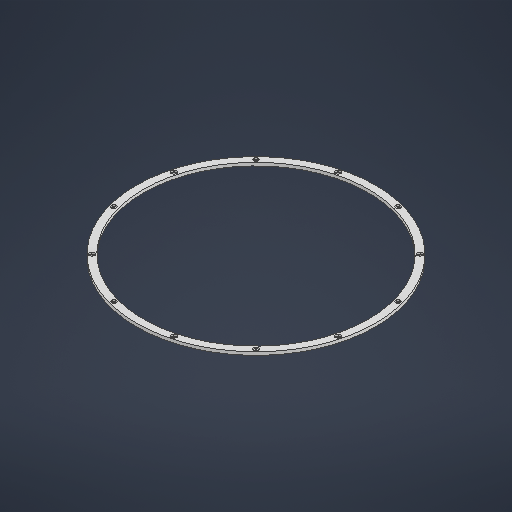
# Autodesk Inventor part: ArmLoopOuterRing
Saved by Autodesk Inventor 2026.1 (Build 301233020, 233B)
## iProperties
Created: 2025-10-19
Part Number: ArmLoopOuterRing
Material: Generic
Document SubType Name: Modeling
Designer: skybound
Density: 1 g/cm^3
Appearance: Default
Author: skybound
Autodesk Inventor part; units mm, degrees
ref_plane "YZ Plane" through (0, 0, 0) normal (1, 0, 0) x (0, 1, 0)
ref_plane "XZ Plane" through (0, 0, 0) normal (0, 1, 0) x (-1, 0, 0)
ref_plane "XY Plane" through (0, 0, 0) normal (0, 0, 1) x (1, 0, 0)
sketch "Sketch1" plane through (0, 0, 0) normal (0, 1, 0) x (-1, 0, 0)
  circle A0 centre (0, 0) radius 144.3
  circle A1 centre (0, 0) radius 153.3
  dimension "d1" = 9
  dimension "d5" = 306.6
  constraints: 2 centre point, 1 coincident
  measures "d1" radial gap between concentric circles of A0 A1
  measures "d5" diameter of A1
extrude "Extrusion1" add sketch "Sketch1" along normal blind 4
sketch "Sketch2" plane through (0, 4, 0) normal (0, 1, 0) x (1, 0, 0)
  line L0 (0, 0) -> (143.7298, 38.5123) construction
  line L1 (146.1384, 40.9209) -> (147.0201, 37.6306)
  line L2 (147.0201, 37.6306) -> (144.6114, 35.222)
  line L3 (144.6114, 35.222) -> (141.3211, 36.1036)
  line L4 (141.3211, 36.1036) -> (140.4395, 39.3939)
  line L5 (140.4395, 39.3939) -> (142.8481, 41.8026)
  line L6 (142.8481, 41.8026) -> (146.1384, 40.9209)
  line L7 (0, 0) -> (153.3, 0) construction
  circle A0 centre (0, 0) radius 153.3 projected
  line L8 (102.8088, 107.6262) -> (106.0991, 108.5078)
  line L9 (101.9272, 104.3359) -> (102.8088, 107.6262)
  line L10 (104.3359, 101.9272) -> (101.9272, 104.3359)
  line L11 (107.6262, 102.8088) -> (104.3359, 101.9272)
  line L12 (108.5078, 106.0991) -> (107.6262, 102.8088)
  line L13 (106.0991, 108.5078) -> (108.5078, 106.0991)
  line L14 (35.222, 144.6114) -> (37.6306, 147.0201)
  line L15 (36.1036, 141.3211) -> (35.222, 144.6114)
  line L16 (39.3939, 140.4395) -> (36.1036, 141.3211)
  line L17 (41.8026, 142.8481) -> (39.3939, 140.4395)
  line L18 (40.9209, 146.1384) -> (41.8026, 142.8481)
  line L19 (37.6306, 147.0201) -> (40.9209, 146.1384)
  line L20 (-41.8026, 142.8481) -> (-40.9209, 146.1384)
  line L21 (-39.3939, 140.4395) -> (-41.8026, 142.8481)
  line L22 (-36.1036, 141.3211) -> (-39.3939, 140.4395)
  line L23 (-35.222, 144.6114) -> (-36.1036, 141.3211)
  line L24 (-37.6306, 147.0201) -> (-35.222, 144.6114)
  line L25 (-40.9209, 146.1384) -> (-37.6306, 147.0201)
  line L26 (-107.6262, 102.8088) -> (-108.5078, 106.0991)
  line L27 (-104.3359, 101.9272) -> (-107.6262, 102.8088)
  line L28 (-101.9272, 104.3359) -> (-104.3359, 101.9272)
  line L29 (-102.8088, 107.6262) -> (-101.9272, 104.3359)
  line L30 (-106.0991, 108.5078) -> (-102.8088, 107.6262)
  line L31 (-108.5078, 106.0991) -> (-106.0991, 108.5078)
  line L32 (-144.6114, 35.222) -> (-147.0201, 37.6306)
  line L33 (-141.3211, 36.1036) -> (-144.6114, 35.222)
  line L34 (-140.4395, 39.3939) -> (-141.3211, 36.1036)
  line L35 (-142.8481, 41.8026) -> (-140.4395, 39.3939)
  line L36 (-146.1384, 40.9209) -> (-142.8481, 41.8026)
  line L37 (-147.0201, 37.6306) -> (-146.1384, 40.9209)
  line L38 (-142.8481, -41.8026) -> (-146.1384, -40.9209)
  line L39 (-140.4395, -39.3939) -> (-142.8481, -41.8026)
  line L40 (-141.3211, -36.1036) -> (-140.4395, -39.3939)
  line L41 (-144.6114, -35.222) -> (-141.3211, -36.1036)
  line L42 (-147.0201, -37.6306) -> (-144.6114, -35.222)
  line L43 (-146.1384, -40.9209) -> (-147.0201, -37.6306)
  line L44 (-102.8088, -107.6262) -> (-106.0991, -108.5078)
  line L45 (-101.9272, -104.3359) -> (-102.8088, -107.6262)
  line L46 (-104.3359, -101.9272) -> (-101.9272, -104.3359)
  line L47 (-107.6262, -102.8088) -> (-104.3359, -101.9272)
  line L48 (-108.5078, -106.0991) -> (-107.6262, -102.8088)
  line L49 (-106.0991, -108.5078) -> (-108.5078, -106.0991)
  line L50 (-35.222, -144.6114) -> (-37.6306, -147.0201)
  line L51 (-36.1036, -141.3211) -> (-35.222, -144.6114)
  line L52 (-39.3939, -140.4395) -> (-36.1036, -141.3211)
  line L53 (-41.8026, -142.8481) -> (-39.3939, -140.4395)
  line L54 (-40.9209, -146.1384) -> (-41.8026, -142.8481)
  line L55 (-37.6306, -147.0201) -> (-40.9209, -146.1384)
  line L56 (41.8026, -142.8481) -> (40.9209, -146.1384)
  line L57 (39.3939, -140.4395) -> (41.8026, -142.8481)
  line L58 (36.1036, -141.3211) -> (39.3939, -140.4395)
  line L59 (35.222, -144.6114) -> (36.1036, -141.3211)
  line L60 (37.6306, -147.0201) -> (35.222, -144.6114)
  line L61 (40.9209, -146.1384) -> (37.6306, -147.0201)
  line L62 (107.6262, -102.8088) -> (108.5078, -106.0991)
  line L63 (104.3359, -101.9272) -> (107.6262, -102.8088)
  line L64 (101.9272, -104.3359) -> (104.3359, -101.9272)
  line L65 (102.8088, -107.6262) -> (101.9272, -104.3359)
  line L66 (106.0991, -108.5078) -> (102.8088, -107.6262)
  line L67 (108.5078, -106.0991) -> (106.0991, -108.5078)
  line L68 (144.6114, -35.222) -> (147.0201, -37.6306)
  line L69 (141.3211, -36.1036) -> (144.6114, -35.222)
  line L70 (140.4395, -39.3939) -> (141.3211, -36.1036)
  line L71 (142.8481, -41.8026) -> (140.4395, -39.3939)
  line L72 (146.1384, -40.9209) -> (142.8481, -41.8026)
  line L73 (147.0201, -37.6306) -> (146.1384, -40.9209)
  dimension "d6" = 148.8
  dimension "d7" = 5.9
  dimension "d8" = 15
  dimension "d11" = 360
  constraints: 148 end point, 1 coincident, 1 horizontal, 1 horizontal alignment, 1 perpendicular, 159 other
  measures "d6" distance of L0.start L0.end
  measures "d7" distance between parallel lines of L1 L4
  measures "d8" angle of L7 L0
extrude "Extrusion2" cut sketch "Sketch2" against normal blind 2 contours L1 L2 L3 L4 L5 L6 | L8 L13 L12 L11 L10 L9 | L14 L19 L18 L17 L16 L15 | L20 L25 L24 L23 L22 L21 | L26 L31 L30 L29 L28 L27 | L32 L37 L36 L35 L34 L33 | L38 L43 L42 L41 L40 L39 | L44 L49 L48 L47 L46 L45 | L50 L55 L54 L53 L52 L51 | L56 L61 L60 L59 L58 L57 | L62 L67 L66 L65 L64 L63 | L68 L73 L72 L71 L70 L69
sketch "Sketch3" plane through (0, 2, 0) normal (0, 1, 0) x (1, 0, 0)
  circle A0 centre (143.7298, 38.5123) radius 1.7
  line L0 (144.6114, 35.222) -> (141.3211, 36.1036) projected
  line L1 (142.8481, 41.8026) -> (146.1384, 40.9209) projected
  line L2 (144.6114, 35.222) -> (142.8481, 41.8026) construction
  circle A1 centre (105.2175, 105.2175) radius 1.7
  circle A2 centre (38.5123, 143.7298) radius 1.7
  circle A3 centre (-38.5123, 143.7298) radius 1.7
  circle A4 centre (-105.2175, 105.2175) radius 1.7
  circle A5 centre (-143.7298, 38.5123) radius 1.7
  circle A6 centre (-143.7298, -38.5123) radius 1.7
  circle A7 centre (-105.2175, -105.2175) radius 1.7
  circle A8 centre (-38.5123, -143.7298) radius 1.7
  circle A9 centre (38.5123, -143.7298) radius 1.7
  circle A10 centre (105.2175, -105.2175) radius 1.7
  circle A11 centre (143.7298, -38.5123) radius 1.7
  point P0 (0, 0)
  dimension "d15" = 3.4
  dimension "d18" = 360
  constraints: 12 centre point, 2 end point, 2 midpoint, 25 other
  measures "d15" diameter of A0
extrude "Extrusion3" cut sketch "Sketch3" against normal through all
body "Solid1"
